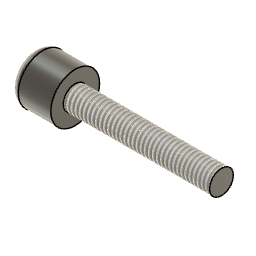
chuck bolt v4 (Autodesk Fusion 360 design; units mm, degrees)
Autodesk Fusion 360 part; units mm, degrees
sketch "草图1" plane through (0, 0, 0) normal (1, 0, 0) x (0, 1, 0)
  circle A0 centre (0, 0) radius 2.5
  dimension "d1" = 5
  constraint coincident A0.centre origin
  measures "d1" diameter of A0
sketch "草图2" plane through (0, 0, 0) normal (-1, 0, 0) x (0, -1, 0)
  circle A0 centre (0, 0) radius 2.5
  circle A1 centre (0, 0) radius 1.5
  dimension "d4" = 3
  constraint concentric A0 A1
  measures "d4" diameter of A1
sketch "草图3" plane through (0, 0, 0) normal (1, 0, 0) x (0, 1, 0)
  circle A0 centre (25, 10) radius 1.5
  dimension "d7" = 3
  measures "d7" diameter of A0
extrude "拉伸3" add sketch "草图3" along normal blind 18
sketch "草图4" plane through (0, 0, 0) normal (-1, 0, 0) x (0, -1, 0)
  circle A0 centre (-25, 10) radius 1.5
  circle A1 centre (-25, 10) radius 3
  dimension "d10" = 6
  constraint concentric A0 A1
  measures "d10" diameter of A1
extrude "拉伸4" add sketch "草图4" along normal blind 5 contours A0 | A1
fillet "圆角1" radius 1 1 edges at (-5, 27.797, 8.9152)
thread "螺纹1" "ISO Metric profile 3.0 M3x0.5 6g" major diameter 2.927 minor diameter 2.3555 pitch 0.5 angle 60 resizes the face on face at (12, 26.4981, 9.9252)
sketch "草图5" plane through (0, 0, 0) normal (0, 0, 1) x (1, 0, 0)
  line L0 (0, 2) -> (7, 2)
  line L1 (10, 2.4683) -> (10, 3.4683)
  line L2 (7, 3.4683) -> (7, 2.4683)
  line L3 (10, 2.4683) -> (7, 2.4683)
  line L4 (7, 2.4683) -> (7, 3.4683)
  line L5 (7, 3.4683) -> (10, 3.4683)
  line L6 (10, 3.4683) -> (10, 2.4683)
  dimension "d15" = 7
  dimension "d16" = 1
  constraint horizontal L0
  constraint vertical L1
  constraint vertical L2
  constraint perpendicular L2 L3
  constraint perpendicular L3 L4
  constraint perpendicular L1 L5
  measures "d15" distance of L0.start L0.end
  measures "d16" distance of L2.end L2.start
sketch "草图6" plane through (0, 0, 0) normal (0, 0, 1) x (1, 0, 0)
  line L0 (0, 0) -> (107, 0)
  constraint coincident L0.start origin
  constraint horizontal L0
sketch "草图7" plane through (107, 0, 0) normal (1, 0, 0) x (0, 1, 0)
  circle A0 centre (0, 0) radius 2.5
  circle A1 centre (0, 0) radius 3
  dimension "d24" = 6
  constraint coincident A0.centre A1.centre
  measures "d24" diameter of A1
sketch "草图8" plane through (117, 0, 0) normal (1, 0, 0) x (0, 1, 0)
  circle A0 centre (0, 0) radius 3
sketch "草图9" plane through (117, 0, 0) normal (1, 0, 0) x (0, 1, 0)
  circle A0 centre (0, 0) radius 2.5
  dimension "d27" = 5
  constraint coincident A0.centre origin
  measures "d27" diameter of A0
sketch "草图10" plane through (207, 0, 0) normal (1, 0, 0) x (0, 1, 0)
  circle A0 centre (0, 0) radius 2.5
  circle A1 centre (0, 0) radius 3
  dimension "d30" = 6
  constraint concentric A0 A1
  measures "d30" diameter of A1
sketch "草图11" plane through (113.9621, 0, 0) normal (1, 0, 0) x (0, 1, 0)
  circle A0 centre (-1.8406, 12.5634) radius 0.75
  circle A1 centre (-4.3473, 13.0634) radius 1
  line L0 (-1.8406, 13.5634) -> (-3.8406, 15.5634)
  line L1 (-3.8406, 15.5634) -> (-6.8406, 15.5634)
  line L2 (-6.8406, 15.5634) -> (-6.8406, 12.5634)
  line L3 (-6.8406, 12.5634) -> (-4.8406, 10.5634)
  line L4 (-4.8406, 10.5634) -> (-2.8406, 10.5634)
  line L5 (-2.8406, 10.5634) -> (-1.8406, 11.5634)
  arc A2 (-1.8406, 11.5634) -> (-1.8406, 13.5634) centre (-1.8406, 12.5634) ccw
  circle A3 centre (-1.8406, 12.5634) radius 0.75
  constraint concentric A0 A3
sketch "草图12" plane through (114.4621, 0, 0) normal (1, 0, 0) x (0, 1, 0)
  circle A0 centre (-1.8406, 12.5634) radius 0.75
  line L0 (-4.3422, 28.7406) -> (-4.5, 29.5)
  line L1 (-5.6584, 28.7421) -> (-2.826, 12.3927)
  line L2 (-4.3422, 28.7406) -> (-0.9157, 12.9436)
  arc A1 (-2.826, 12.3927) -> (-0.9157, 12.9436) centre (-1.8406, 12.5634) ccw
  arc A2 (-4.3422, 28.7406) -> (-5.6584, 28.7421) centre (-5, 29) ccw
  dimension "d49" = 2
  constraint concentric A0 A1
  constraint tangent L1 A1
  measures "d49" diameter of A1
sketch "草图13" plane through (114.4621, 0, 0) normal (-1, 0, 0) x (0, -1, 0)
  line L0 (4.5, 29.5) -> (4.3422, 28.7406)
  line L1 (4.3422, 28.7406) -> (0.9157, 12.9436)
  arc A0 (0.9157, 12.9436) -> (2.826, 12.3927) centre (1.8406, 12.5634) ccw
  line L2 (2.826, 12.3927) -> (5.6584, 28.7421)
  arc A1 (5.6584, 28.7421) -> (4.5, 29.5) centre (5, 29) ccw
  circle A2 centre (1.8406, 12.5634) radius 0.75
sketch "草图14" plane through (111.3616, -5.0975, 0) normal (-0.998954, 0.045726, 0) x (-0.045726, -0.998954, 0)
  arc A0 (-0.6828, 29.5605) -> (0.4235, 28.5491) centre (-0.1488, 29.0338) ccw
  line L0 (0.4235, 28.5491) -> (5.7118, 34.0644)
  arc A1 (4.7121, 35.0312) -> (5.7118, 34.0644) centre (5.7115, 35.0644) ccw
  line L1 (4.7121, 35.0312) -> (-0.6828, 29.5605)
sketch "草图15" plane through (115.3574, -5.2804, 0) normal (0.998954, -0.045726, 0) x (0.045726, 0.998954, 0)
  arc A0 (-0.4235, 28.5491) -> (0.6828, 29.5605) centre (0.1488, 29.0338) ccw
  line L0 (0.6828, 29.5605) -> (-4.7121, 35.0312)
  arc A1 (-5.7118, 34.0644) -> (-4.7121, 35.0312) centre (-5.7115, 35.0644) ccw
  line L1 (-5.7118, 34.0644) -> (-0.4235, 28.5491)
  line L2 (-4, 34) -> (-4.7218, 33.3079)
  line L3 (-4.7218, 33.3079) -> (-1.716, 30.1731)
  line L4 (-1.716, 30.1731) -> (-0.9942, 30.8652)
  line L5 (-0.9942, 30.8652) -> (-4, 34)
  dimension "d72" = 1
  dimension "d73" = 1
  constraint perpendicular L1 L2
  constraint perpendicular L2 L3
  constraint perpendicular L3 L4
  measures "d72" distance of L2.start L2.end
  measures "d73" distance of L3.end L4.end
extrude "拉伸13" [suppressed]
sketch "草图16" plane through (213.9621, 0, 0) normal (1, 0, 0) x (0, 1, 0)
  circle A0 centre (-1.8406, 12.5634) radius 0.75
  circle A1 centre (-4.3473, 13.0634) radius 1
  line L0 (-1.8406, 13.5634) -> (-3.8406, 15.5634)
  line L1 (-3.8406, 15.5634) -> (-6.8406, 15.5634)
  line L2 (-6.8406, 15.5634) -> (-6.8406, 12.5634)
  line L3 (-6.8406, 12.5634) -> (-4.8406, 10.5634)
  line L4 (-4.8406, 10.5634) -> (-2.8406, 10.5634)
  line L5 (-2.8406, 10.5634) -> (-1.8406, 11.5634)
  arc A2 (-1.8406, 11.5634) -> (-1.8406, 13.5634) centre (-1.8406, 12.5634) ccw
  circle A3 centre (-1.8406, 12.5634) radius 0.75
  constraint concentric A0 A3
sketch "草图17" plane through (213.9621, 0, 0) normal (1, 0, 0) x (0, 1, 0)
  circle A0 centre (-1.8406, 12.5634) radius 0.75
  line L0 (-2.8375, 12.4848) -> (-2.8375, 33.2416)
  line L1 (-0.8555, 12.7353) -> (-1.2658, 33.0212)
  arc A1 (-1.2658, 33.0212) -> (-2.8375, 33.2416) centre (-2, 33.5) ccw
  arc A2 (-2.8375, 12.6419) -> (-0.8555, 12.7353) centre (-1.8406, 12.5634) ccw
  dimension "d79" = 2
  constraint concentric A0 A2
  constraint coincident L0.start A2
  constraint vertical L0
  constraint coincident L0 A2.start
  measures "d79" diameter of A2
sketch "草图18" plane through (212.9621, 0, 0) normal (1, 0, 0) x (0, 1, 0)
  circle A0 centre (-10.8473, 60.0634) radius 0.75
  line L0 (-11.3473, 61.5634) -> (-11.3473, 60.9294)
  arc A1 (-11.3473, 60.9294) -> (-10.3473, 60.9294) centre (-10.8473, 60.0634) ccw
  line L1 (-10.3473, 60.9294) -> (-10.3473, 61.5634)
  line L2 (-10.3473, 61.5634) -> (-11.3473, 61.5634)
  line L3 (-11.519, 59.3225) -> (-9.373, 49.2871)
  line L4 (-9.8476, 60.041) -> (-7.3998, 49.4689)
  arc A2 (-9.8476, 60.041) -> (-11.519, 59.3225) centre (-10.8473, 60.0634) ccw
  arc A3 (-9.373, 49.2871) -> (-7.3998, 49.4689) centre (-8.374, 49.2433) ccw
  dimension "d86" = 2
  constraint concentric A0 A2
  constraint coincident A1 L3.start
  constraint tangent L4 A3
  measures "d86" diameter of A3
sketch "草图19" plane through (217, 0, 0) normal (1, 0, 0) x (0, 1, 0)
  circle A0 centre (0, 0) radius 3
  circle A1 centre (0, 0) radius 3
  constraint concentric A0 A1
sketch "草图20" plane through (237, 0, 0) normal (1, 0, 0) x (0, 1, 0)
  circle A0 centre (0, 0) radius 3
  line L0 (-1, 3.5) -> (1, 3.5)
  line L1 (1, 3.5) -> (1, -3.5)
  line L2 (1, -3.5) -> (-1, -3.5)
  line L3 (-1, -3.5) -> (-1, 3.5)
  line L4 (-1, 3.5) -> (1, -3.5) construction
  line L5 (1, 3.5) -> (-1, -3.5) construction
  constraint horizontal L0
  constraint perpendicular L0 L1
  constraint parallel L0 L2
  constraint parallel L1 L3
  constraint coincident L4 A0.centre
  constraint coincident L5 A0.centre
  constraint coincident A0.centre origin
